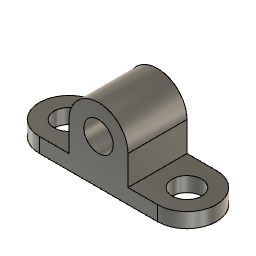
A4 (Autodesk Fusion 360 design; units mm, degrees)
Autodesk Fusion 360 part; units mm, degrees
sketch "Sketch1" plane through (0, 0, 0) normal (0, 0, 1) x (1, 0, 0)
  line L0 (80, 40) -> (0, 40)
  arc A0 (0, 40) -> (0, 0) centre (0, 20) ccw
  arc A1 (80, 0) -> (80, 40) centre (80, 20) ccw
  line L1 (0, 0) -> (80, 0)
  constraint horizontal L0
  constraint tangent L0 A1
  constraint tangent A1 L1
extrude "Extrude1" add sketch "Sketch1" along normal blind 10
hole "Hole1" at (0, 20, 10) direction (0, 0, -1) diameter 20 depth 20 tip angle 118
hole "Hole2" at (80, 20, 10) direction (0, 0, -1) diameter 20 depth 20 tip angle 118
sketch "Sketch2" plane through (0, 0, 0) normal (0, 0, 1) x (1, 0, 0)
  line L0 (20, 0) -> (60, 0)
  line L1 (60, 0) -> (60, 40)
  line L2 (60, 40) -> (20, 40)
  line L3 (20, 40) -> (20, 0)
  constraint horizontal L0
  constraint vertical L1
  constraint horizontal L2
  constraint vertical L3
extrude "Extrude2" add sketch "Sketch2" along normal blind 30
sketch "Sketch3" plane through (0, 0, 0) normal (0, 1, 0) x (1, 0, 0)
  line L0 (60, -30) -> (20, -30)
  arc A0 (20, -30) -> (60, -30) centre (40, -30) ccw
extrude "Extrude3" add sketch "Sketch3" along normal blind 40
hole "Hole3" at (40, 0, 30) direction (0, 1, 0) diameter 20 depth 40 tip angle 118
named bodies: "A4"
